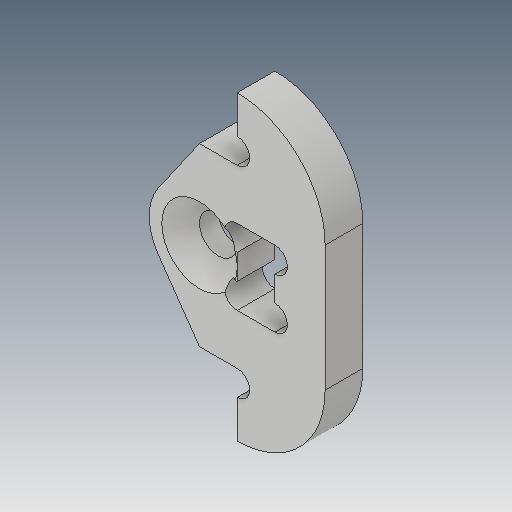
# Autodesk Inventor part: ShaftBase2
Saved by Autodesk Inventor 2019.4 (Build 234330000, 330)
## iProperties
Created: 2019-06-11
Part Number: ShaftBase2
Material: Generic
Document SubType Name: Modeling
Designer: AzLIer
Density: 1 g/cm^3
Appearance: Default
Author: AzLIer
Autodesk Inventor part; units mm, degrees
ref_plane "YZ Plane" through (0, 0, 0) normal (1, 0, 0) x (0, 1, 0)
ref_plane "XZ Plane" through (0, 0, 0) normal (0, 1, 0) x (-1, 0, 0)
ref_plane "XY Plane" through (0, 0, 0) normal (0, 0, 1) x (1, 0, 0)
sketch "スケッチ5" plane through (0, 0, 0) normal (0, 0, 1) x (1, 0, 0)
  line L0 (-1, 1) -> (-1, -1)
  circle A0 centre (-4, 0) radius 1.5
  arc A1 (2, 1) -> (2, 3) centre (2, 2) ccw
  arc A2 (2, -3) -> (2, -1) centre (2, -2) ccw
  arc A3 (-1, 3) -> (-1, 1) centre (-1, 2) ccw
  arc A4 (-1, -1) -> (-1, -3) centre (-1, -2) ccw
  line L1 (2, -3) -> (-1, -3)
  line L2 (-1, 3) -> (2, 3)
  arc A5 (-7.2826, 2.2857) -> (-7.2826, -2.2857) centre (-4, 0) ccw
  line L3 (-1, -7) -> (-1, -7)
  line L4 (6, -5) -> (6, 5)
  line L5 (-1, 7) -> (-1, 7)
  line L6 (0, 0) -> (-1, 0) construction
  arc A6 (-1, -9) -> (-1, -7) centre (-1, -8) ccw
  line L7 (-1, -9) -> (-1, -12)
  arc A7 (-1, -12) -> (6, -5) centre (-1, -5) ccw
  arc A8 (6, 5) -> (-1, 12) centre (-1, 5) ccw
  line L8 (-1, 12) -> (-1, 9)
  arc A9 (-1, 7) -> (-1, 9) centre (-1, 8) ccw
  line L9 (2, -1) -> (2, 1)
  line L10 (-7.2826, -2.2857) -> (-4, -7)
  line L11 (-4, -7) -> (-1, -7)
  line L12 (-7.2826, 2.2857) -> (-4, 7)
  line L13 (-4, 7) -> (-1, 7)
  point P0 (2, 0)
  point P1 (6, 0)
  point P2 (2, 0)
  dimension "d57" = 3
  dimension "d58" = 2
  dimension "d60" = 4
  dimension "d61" = 4
  dimension "d62" = 3
  dimension "d63" = 14
  dimension "d65" = 4
  dimension "d66" = 3
  dimension "d67" = 2
  dimension "d68" = 3
  dimension "d69" = 6
  dimension "d72" = 3
  constraints: 28 end point, 18 point on circle, 11 point on line, 10 centre point, 6 equal radius, 5 tangent, 4 horizontal, 3 equal length, 3 horizontal alignment, 3 midpoint, 2 coincident, 2 parallel, 2 vertical, 1 collinear, 1 perpendicular, 2 other
  measures "d57" diameter of A0
  measures "d58" diameter of A1
  measures "d60" distance of L6.start A0.centre
  measures "d61" radius of A5
  measures "d62" horizontal distance of L5.end A0.centre
  measures "d63" distance between parallel lines of L5 L3
  measures "d65" distance from line of point (2, 0) L4
  measures "d66" distance of L7.start L7.end
  measures "d67" distance from line of L6.start L9
  measures "d68" distance between parallel lines of L9 L0
  measures "d69" distance between parallel lines of L2 L1
  measures "d72" distance of L12.end L5.start
extrude "押し出し2" add sketch "スケッチ5" along normal blind 3
chamfer "面取り2" distance 1.5 angle 45 1 edges at (-5.5, 0, 3)
